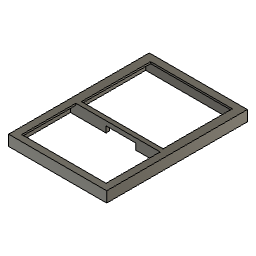
frame (Autodesk Fusion 360 design; units mm, degrees)
Autodesk Fusion 360 part; units mm, degrees
sketch "Sketch1" plane through (0, 0, 0) normal (0, 0, 1) x (1, 0, 0)
  line L0 (3.5, 81.3196) -> (3.5, -80.4746) construction
  line L1 (55.75, 77.2981) -> (-48.75, 77.2981)
  line L2 (-48.75, 77.2981) -> (-48.75, -2.2019)
  line L3 (-48.75, -2.2019) -> (55.75, -2.2019)
  line L4 (55.75, -2.2019) -> (55.75, 77.2981)
  line L5 (55.75, 77.2981) -> (-48.75, -2.2019) construction
  line L6 (-48.75, 77.2981) -> (55.75, -2.2019) construction
  line L7 (-44, -6.2019) -> (51, -6.2019)
  line L8 (51, -6.2019) -> (51, -67.2019)
  line L9 (51, -67.2019) -> (-44, -67.2019)
  line L10 (-44, -67.2019) -> (-44, -6.2019)
  line L11 (-44, -6.2019) -> (51, -67.2019) construction
  line L12 (51, -6.2019) -> (-44, -67.2019) construction
  line L13 (-42.5, 76.5481) -> (49.5, 76.5481)
  line L14 (49.5, 76.5481) -> (49.5, -1.4519)
  line L15 (49.5, -1.4519) -> (-42.5, -1.4519)
  line L16 (-42.5, -1.4519) -> (-42.5, 76.5481)
  line L17 (-42.5, 76.5481) -> (49.5, -1.4519) construction
  line L18 (49.5, 76.5481) -> (-42.5, -1.4519) construction
  line L19 (57, -6.2019) -> (-50, -6.2019)
  line L20 (-50, -6.2019) -> (-50, -67.2019)
  line L21 (-50, -67.2019) -> (57, -67.2019)
  line L22 (57, -67.2019) -> (57, -6.2019)
  line L23 (57, -6.2019) -> (-50, -67.2019) construction
  line L24 (-50, -6.2019) -> (57, -67.2019) construction
  line L25 (-209.3085, -13.7554) -> (162.3486, -13.7554) construction
  line L26 (58.75, -74.2019) -> (-51.75, -74.2019)
  line L27 (-51.75, -74.2019) -> (-51.75, 84.2981)
  line L28 (-51.75, 84.2981) -> (58.75, 84.2981)
  line L29 (58.75, 84.2981) -> (58.75, -74.2019)
  line L30 (58.75, -74.2019) -> (-51.75, 84.2981) construction
  line L31 (-51.75, -74.2019) -> (58.75, 84.2981) construction
  line L32 (-9.9758, -6.2019) -> (23.4575, -6.2019)
  line L33 (23.4575, -6.2019) -> (23.4575, -1.4519)
  line L34 (23.4575, -1.4519) -> (-9.9758, -1.4519)
  line L35 (-9.9758, -1.4519) -> (-9.9758, -6.2019)
  point P0 (3.5, 37.5481)
  point P1 (3.5, -36.7019)
  point P2 (3.5, 37.5481)
  point P3 (3.5, -36.7019)
  point P4 (3.5, 5.0481)
  dimension "d11" = 104.5
  dimension "d12" = 79.5
  dimension "d13" = 95
  dimension "d14" = 61
  dimension "d15" = 92
  dimension "d16" = 78
  dimension "d17" = 107
  dimension "d18" = 61
  dimension "d19" = 74.25
  dimension "d21" = 110.5
  dimension "d22" = 158.5
  dimension "d23" = 7
  constraint vertical L0
  constraint horizontal L1
  constraint perpendicular L1 L2
  constraint parallel L1 L3
  constraint parallel L2 L4
  constraint coincident L5 P2
  constraint coincident L6 P2
  constraint coincident L0 P2
  constraint horizontal L7
  constraint perpendicular L7 L8
  constraint parallel L7 L9
  constraint parallel L8 L10
  constraint coincident L11 P3
  constraint coincident L12 P3
  constraint coincident L0 P3
  constraint horizontal L13
  constraint perpendicular L13 L14
  constraint parallel L13 L15
  constraint parallel L14 L16
  constraint coincident L17 P2
  constraint coincident L18 P2
  constraint coincident P2 P0
  constraint horizontal L19
  constraint perpendicular L19 L20
  constraint parallel L19 L21
  constraint parallel L20 L22
  constraint coincident L23 P3
  constraint coincident L24 P3
  constraint coincident P3 P1
  constraint perpendicular L4 L25
  constraint horizontal L26
  constraint perpendicular L26 L27
  constraint parallel L26 L28
  constraint parallel L27 L29
  constraint coincident L30 P4
  constraint coincident L31 P4
  constraint coincident L0 P4
  constraint horizontal L32
  constraint vertical L33
  constraint horizontal L34
  constraint vertical L35
  constraint coincident L15 L33.end
  constraint coincident L19 L32.start
  measures "d11" distance of L2.end L3.end
  measures "d12" distance of L1.end L2.end
  measures "d13" distance of L8.end L9.end
  measures "d14" distance of L7.end L8.end
  measures "d15" distance of L14.end L15.end
  measures "d16" distance of L13.end L14.end
  measures "d17" distance of L20.end L21.end
  measures "d18" distance of L19.end L20.end
  measures "d19" distance of P2 P3
  measures "d21" distance of L27.end L28.end
  measures "d22" distance of L26.end L27.end
  measures "d23" distance of L1 L28
extrude "Extrude1" add sketch "Sketch1" along normal blind 2 contours L1 L2 L3 L4 L13 L14 L15 L16 L33 L35 | L3 L7 L19 L32 L33 L35 | L3 L15 L33 L34 L35 | L8 L19 L21 L22 | L10 L19 L20 L21 | L26 L27 L28 L29
extrude "Extrude2" add sketch "Sketch1" against normal blind 10
extrude "Extrude3" add sketch "Sketch1" against normal blind 3 contours L3 L7 L19 L32 L33 L35
equation "screenWidth = 92 mm"
equation "screenHeight = 78 mm"
equation "solarWidth = 107 mm"
equation "solarHeight = 61 mm"
equation "solarBoardWidth = 95 mm"
equation "solarBoardOHeight = solarHeight"
equation "screenBoardWidth = 104.5 mm"
equation "screenBoardHeight = 79.5 mm"
equation "middleSpace = 4 mm"
equation "border = 3 mm"
equation "d11 = screenBoardWidth"
equation "d12 = screenBoardHeight"
equation "d13 = solarBoardWidth"
equation "d14 = solarBoardOHeight"
equation "d15 = screenWidth"
equation "d16 = screenHeight"
equation "d17 = solarWidth"
equation "d18 = solarHeight"
equation "d19 = ( ( screenBoardHeight + solarBoardOHeight ) / 2 ) + middleSpace"
equation "boardThickness = 10 mm"
equation "d21 = screenBoardWidth + ( border * 2 )"
equation "d22 = solarBoardOHeight + screenBoardHeight + middleSpace + ( borderTop * 2 )"
equation "d23 = borderTop"
equation "faceThickness = 2 mm"
equation "d25 = faceThickness"
equation "d27 = -boardThickness"
equation "borderTop = 7 mm"
